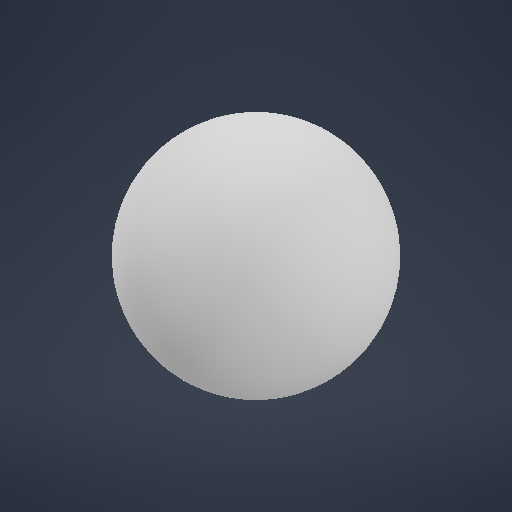
# Autodesk Inventor part: esfera20
Saved by Autodesk Inventor 2026.3 (Build 303398000, 398)
## iProperties
Created: 2026-05-16
Part Number: esfera20
Material: Genérico
Document SubType Name: Modeling
Designer: alenc
Density: 1 g/cm^3
Appearance: Padrão
Author: alenc
Autodesk Inventor part; units mm, degrees
ref_plane "YZ Plane" through (0, 0, 0) normal (1, 0, 0) x (0, 1, 0)
ref_plane "XZ Plane" through (0, 0, 0) normal (0, 1, 0) x (-1, 0, 0)
ref_plane "XY Plane" through (0, 0, 0) normal (0, 0, 1) x (1, 0, 0)
sketch "Esboço1" plane through (0, 0, 0) normal (0, 0, 1) x (1, 0, 0)
  arc A0 (10, 0) -> (-10, 0) centre (0, 0) ccw
  line L0 (-10, 0) -> (10, 0)
  dimension "d0" = 20
  constraints: 2 end point, 2 point on circle, 1 centre point, 1 coincident, 1 horizontal
  measures "d0" distance of L0.start L0.end
revolve "Revolução1" add sketch "Esboço1" angle 360 about axis through (-10, 0, 0) along (1, 0, 0)
